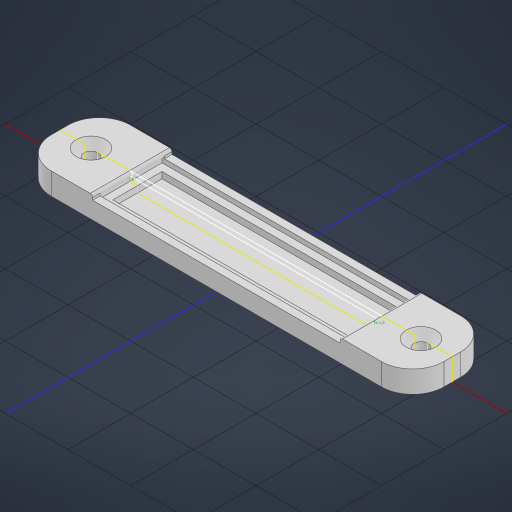
# Autodesk Inventor part: PCB_Holder_A
Saved by Autodesk Inventor 2023.2 (Build 272271030, 271C)
## iProperties
Created: 2023-05-22
Part Number: PCB_Holder_A
Material: Generisch
Document SubType Name: Modeling
Designer: Stefan
Mass: 13.3966 g
Surface Area: 88.1579 cm^2
Volume: 13.3966 cm^3
Density: 1 g/cm^3
Appearance: Vorgabe
Author: Stefan
Autodesk Inventor part; units mm, degrees
ref_plane "YZ Plane" through (0, 0, 0) normal (1, 0, 0) x (0, 1, 0)
ref_plane "XZ Plane" through (0, 0, 0) normal (0, 1, 0) x (-1, 0, 0)
ref_plane "XY Plane" through (0, 0, 0) normal (0, 0, 1) x (1, 0, 0)
sketch "Skizze1" plane through (0, 0, 0) normal (0, 1, 0) x (-1, 0, 0)
  line L0 (40.25, -10.25) -> (-40.25, -10.25)
  line L1 (-40.25, -10.25) -> (-40.25, 10.25)
  line L2 (-40.25, 10.25) -> (40.25, 10.25)
  line L3 (40.25, 10.25) -> (40.25, -10.25)
  line L4 (40.25, -10.25) -> (-40.25, 10.25) construction
  line L5 (-40.25, -10.25) -> (40.25, 10.25) construction
  line L6 (42.65, -12.65) -> (-42.65, -12.65)
  line L7 (-42.65, -12.65) -> (-42.65, 12.65)
  line L8 (-42.65, 12.65) -> (42.65, 12.65)
  line L9 (42.65, 12.65) -> (42.65, -12.65)
  line L10 (37.85, -7.85) -> (-37.85, -7.85)
  line L11 (-37.85, -7.85) -> (-37.85, 7.85)
  line L12 (-37.85, 7.85) -> (37.85, 7.85)
  line L13 (37.85, 7.85) -> (37.85, -7.85)
  line L14 (52.65, -12.65) -> (42.65, -12.65)
  line L15 (42.65, 12.65) -> (52.65, 12.65)
  circle A0 centre (52.65, 0) radius 2
  line L16 (-42.65, -12.65) -> (-52.65, -12.65)
  line L17 (-42.65, 12.65) -> (-52.65, 12.65)
  circle A1 centre (-52.65, 0) radius 2
  arc A2 (62.65, 2.65) -> (52.65, 12.65) centre (52.65, 2.65) ccw
  arc A3 (52.65, -12.65) -> (62.65, -2.65) centre (52.65, -2.65) ccw
  line L18 (62.65, 2.65) -> (62.65, -2.65)
  arc A4 (-52.65, 12.65) -> (-62.65, 2.65) centre (-52.65, 2.65) ccw
  arc A5 (-62.65, -2.65) -> (-52.65, -12.65) centre (-52.65, -2.65) ccw
  line L19 (-62.65, 2.65) -> (-62.65, -2.65)
  point P0 (0, 0)
  point P1 (62.65, 0)
  point P2 (-62.65, 0)
  dimension "d0" = 80.5
  dimension "d1" = 20.5
  dimension "d2" = 2.4
  dimension "d3" = 2.4
  dimension "d4" = 4
  dimension "d7" = 4
  dimension "d25" = 20
  dimension "d26" = 10
  dimension "d27" = 10
  dimension "d28" = 20
  dimension "d29" = 10
  dimension "d30" = 10
  constraints: 40 end point, 8 parallel, 8 point on circle, 8 tangent, 6 centre point, 4 collinear, 4 midpoint, 3 perpendicular, 2 equal radius, 2 horizontal alignment, 1 horizontal, 6 other
  measures "d0" distance of L1.end L2.end
  measures "d1" distance of L0.end L1.end
  measures "d2" distance between parallel lines of L3 L9
  measures "d3" distance between parallel lines of L13 L3
  measures "d4" diameter of A0
  measures "d7" diameter of A1
  measures "d25" distance between parallel lines of L18 L9
  measures "d26" radius of A2
  measures "d27" distance from line of L9 A0.centre
  measures "d28" distance between parallel lines of L19 L7
  measures "d29" distance from line of A1.centre L7
  measures "d30" radius of A4
extrude "Extrusion1" add sketch "Skizze1" against normal blind 2 contours L0 L1 L2 L3 | L6 L7 L8 L9 | L9 L15 A2 L18 A3 L14 | L16 A5 L19 A4 L17 L7 | L10 L11 L12 L13
extrude "Extrusion2" add sketch "Skizze1" along normal blind 5 contours L6 L7 L8 L9 | L9 L15 A2 L18 A3 L14 | L16 A5 L19 A4 L17 L7
extrude "Extrusion3" add sketch "Skizze1" along normal blind 2 contours L0 L1 L2 L3
sketch "Skizze2" plane through (0, 0, 0) normal (0, 0, 1) x (1, 0, 0)
  line L0 (37.85, 0) -> (37.85, 2) projected
  line L1 (37.85, 2) -> (40.25, 2) projected
  line L2 (40.25, 2) -> (40.25, 5) projected
  line L3 (40.25, 5) -> (50.65, 5) projected
  line L4 (50.65, 5) -> (50.65, -2) projected
  line L5 (50.65, -2) -> (-50.65, -2) projected
  line L6 (-50.65, -2) -> (-50.65, 5) projected
  line L7 (-50.65, 5) -> (-40.25, 5) projected
  line L8 (-40.25, 5) -> (-40.25, 2) projected
  line L9 (-40.25, 2) -> (-37.85, 2) projected
  line L10 (-37.85, 2) -> (-37.85, 0) projected
  line L11 (-37.85, 0) -> (37.85, 0) projected
  line L12 (-62.65, 5) -> (-54.65, 5) projected
  line L13 (-54.65, 5) -> (-54.65, -2) projected
  line L14 (-54.65, -2) -> (-62.65, -2) projected
  line L15 (54.65, 5) -> (62.65, 5) projected
  line L16 (62.65, -2) -> (54.65, -2) projected
  line L17 (54.65, -2) -> (54.65, 5) projected
  arc A0 (-40.25, 3.5) -> (-40.25, 5) centre (-40.25, 4.25) ccw
  arc A1 (40.25, 5) -> (40.25, 3.5) centre (40.25, 4.25) ccw
  line L18 (-40.25, 5) -> (-40.25, 3.5)
  line L19 (40.25, 5) -> (40.25, 3.5)
  line L20 (-62.65, -2) -> (-62.65, 5) projected
  line L21 (62.65, 5) -> (62.65, -2) projected
  line L22 (-40.25, 3.5) -> (40.25, 3.5)
  line L23 (40.25, 5) -> (-40.25, 5)
  line L24 (-39.5, 4.25) -> (-39.5, 3.5)
  line L25 (39.5, 4.25) -> (39.5, 3.5)
  point P0 (0, 0)
  dimension "d14" = 1.5
  dimension "d15" = 1.5
  constraints: 12 end point, 6 point on circle, 2 centre point, 2 collinear, 2 midpoint, 2 perpendicular, 2 point on line, 2 tangent, 1 vertical
  measures "d14" distance from line of L18.end L9
  measures "d15" distance from line of L19.end L1
extrude "Extrusion4" add sketch "Skizze2" along normal mid plane 20.5 contours A1 L2 | L8 A0
sketch "Skizze3" plane through (0, 5, 0) normal (0, 1, 0) x (1, 0, 0)
  circle A0 centre (-52.65, 0) radius 2 projected
  circle A1 centre (52.65, 0) radius 2 projected
  point P0 (0, 0)
  constraints: 2 coincident
hole "Bohrung1" at (-52.65, 5, 0) at (52.65, 5, 0) direction (0, -1, 0) diameter 4.5 depth 6 countersink diameter 9.4 countersink angle 90 clearance for "Flachkopfsenkschraube DIN EN ISO 2009" size "M4" standard "DIN"
extrude "Extrusion5" cut sketch "Skizze2" along normal through all both and the other way through all contours A1 L25 L22 L24 A0 L23
equation "\"d7\" = d4"
equation "\"d28\" = d25"
equation "\"d29\" = d27"
equation "\"d30\" = d26"
equation "\"d15\" = d14"
